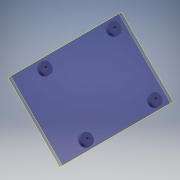
# Autodesk Inventor part: ChassisPrototypeA5
Saved by Autodesk Inventor 2017 (Build 210142000, 142)
## iProperties
Created: 2018-04-24
Part Number: ChassisPrototypeA5
Material: Generic
Document SubType Name: Modeling
Designer: MtgSaber
Mass: 8.35184 g
Surface Area: 62.5115 cm^2
Volume: 8.35184 cm^3
Density: 1 g/cm^3
Appearance: Default
Author: MtgSaber
Autodesk Inventor part; units mm, degrees
ref_plane "YZ Plane" through (0, 0, 0) normal (1, 0, 0) x (0, 1, 0)
ref_plane "Work Plane1" through (108.406, 19.8015, 0) normal (-0.7071068, -0.7071068, 0) x (0, 0, -1)
ref_plane "Work Plane2" through (106.1609, 17.5564, 0) normal (-0.7071068, -0.7071068, 0) x (0, 0, -1)
sketch "Sketch2" plane through (106.1609, 17.5564, 0) normal (-0.7071068, -0.7071068, 0) x (0, 0, -1)
  circle A0 centre (38.989, 24.4983) radius 1.3716 construction
  arc A1 (42.4942, 25.0063) -> (39.497, 28.0035) centre (39.497, 25.0063) ccw construction
  circle A2 centre (38.989, -24.4983) radius 1.3716 construction
  arc A3 (39.497, -28.0035) -> (42.4942, -25.0063) centre (39.497, -25.0063) ccw construction
  circle A4 centre (38.989, 24.4983) radius 1.3716 construction
  circle A5 centre (-18.9992, 24.4983) radius 1.3716 construction
  circle A6 centre (-18.9992, -24.4983) radius 1.3716 construction
  circle A7 centre (38.989, -24.4983) radius 1.3716 construction
  line L0 (-42.4942, 25.0063) -> (-42.4942, -25.0063) construction
  arc A8 (-42.4942, -25.0063) -> (-39.497, -28.0035) centre (-39.497, -25.0063) ccw construction
  line L1 (-39.497, -28.0035) -> (39.497, -28.0035) construction
  arc A9 (39.497, -28.0035) -> (42.4942, -25.0063) centre (39.497, -25.0063) ccw construction
  line L2 (42.4942, -25.0063) -> (42.4942, 25.0063) construction
  arc A10 (42.4942, 25.0063) -> (39.497, 28.0035) centre (39.497, 25.0063) ccw construction
  line L3 (39.497, 28.0035) -> (-39.497, 28.0035) construction
  arc A11 (-39.497, 28.0035) -> (-42.4942, 25.0063) centre (-39.497, 25.0063) ccw construction
  circle A12 centre (38.989, 24.4983) radius 1.3716
  circle A13 centre (38.989, 24.4983) radius 4.5466
  circle A14 centre (38.989, -24.4983) radius 1.3716
  circle A15 centre (38.989, -24.4983) radius 4.5466
  circle A16 centre (-18.9992, -24.4983) radius 1.3716
  circle A17 centre (-18.9992, -24.4983) radius 4.5466
  circle A18 centre (-18.9992, 24.4983) radius 1.3716
  circle A19 centre (-18.9992, 24.4983) radius 4.5466
  point P0 (0, -62.6529)
  dimension "d5" = 3.175
  constraints: 8 centre point, 8 coincident, 7 equal radius
  measures "d5" radial gap between concentric circles of A5 A19
extrude "Extrusion1" add sketch "Sketch2" along normal blind 3.175
ref_plane "Work Plane3" through (127.2196, 3.2509, 0) normal (0, 0, 1) x (-0.7071068, -0.7071068, 0)
sketch "Sketch3" plane through (127.2196, 3.2509, 0) normal (0, 0, 1) x (-0.7071068, -0.7071068, 0)
  line L0 (7.9502, -54.0512) -> (7.9502, -44.958) construction
  line L1 (7.9502, -5.0546) -> (7.9502, 4.0386) construction
  line L2 (7.9502, -54.0512) -> (7.9502, -44.958) construction
  line L3 (7.9502, -54.0512) -> (7.9502, 4.0386) construction
  line L4 (41.241, -25.0063) -> (7.9502, -58.2971) construction
  line L5 (41.241, -25.0063) -> (7.9502, 8.2845) construction
  circle A0 centre (32.2607, -25.0063) radius 2.0574
  arc A1 (36.7508, -29.4964) -> (36.7508, -20.5162) centre (32.2607, -25.0063) ccw
  line L6 (7.9502, -25.0063) -> (55.6437, -25.0063) construction
  circle A2 centre (23.2805, -33.9866) radius 2.0574
  circle A3 centre (23.2805, -33.9866) radius 6.35 construction
  circle A4 centre (14.3002, -7.0458) radius 2.0574
  arc A5 (18.7903, -2.5557) -> (14.3002, -0.6958) centre (14.3002, -7.0458) ccw
  circle A6 centre (23.2805, -16.026) radius 2.0574
  circle A7 centre (23.2805, -16.026) radius 6.35 construction
  circle A8 centre (14.3002, -42.9668) radius 2.0574
  arc A9 (14.3002, -49.3168) -> (18.7903, -47.4569) centre (14.3002, -42.9668) ccw
  circle A10 centre (14.3002, -25.0063) radius 2.0574 construction
  circle A11 centre (14.3002, -25.0063) radius 6.35 construction
  line L7 (7.9502, -42.9668) -> (7.9502, -7.0458)
  line L8 (18.7903, -2.5557) -> (36.7508, -20.5162)
  line L9 (36.7508, -29.4964) -> (18.7903, -47.4569)
  arc A12 (16.3576, -20.8915) -> (12.2428, -20.8915) centre (14.3002, -20.8915) ccw
  line L10 (14.3002, -42.9668) -> (14.3002, -7.0458) construction
  arc A13 (12.2428, -29.1211) -> (16.3576, -29.1211) centre (14.3002, -29.1211) ccw
  arc A14 (18.415, -27.0637) -> (18.415, -22.9489) centre (18.415, -25.0063) ccw
  line L11 (16.3576, -27.0637) -> (18.415, -27.0637)
  line L12 (16.3576, -22.9489) -> (18.415, -22.9489)
  line L13 (16.3576, -27.0637) -> (16.3576, -29.1211)
  line L14 (16.3576, -22.9489) -> (16.3576, -20.8915)
  line L15 (12.2428, -20.8915) -> (12.2428, -29.1211)
  line L16 (14.3002, -49.3168) -> (7.9502, -49.3168)
  line L17 (7.9502, -42.9668) -> (7.9502, -49.3168)
  line L18 (14.3002, -0.6958) -> (7.9502, -0.6958)
  line L19 (7.9502, -0.6958) -> (7.9502, -7.0458)
  point P0 (92.2566, -87.6592)
  dimension "d8" = 45
  dimension "d9" = 4.1148
  dimension "d10" = 12.7
  dimension "d11" = 4.1148
  dimension "d12" = 12.7
  dimension "d13" = 4.1148
  dimension "d14" = 12.7
  dimension "d15" = 4.1148
  dimension "d16" = 12.7
  dimension "d19" = 4.1148
  dimension "d20" = 12.7
  dimension "d21" = 4.1148
  dimension "d22" = 12.7
  dimension "d23" = 4.1148
  dimension "d24" = 4.1148
  dimension "d25" = 4.1148
  constraints: 32 end point, 15 centre point, 13 tangent, 12 point on circle, 10 point on line, 7 equal radius, 6 coincident, 4 parallel, 3 vertical, 2 horizontal, 2 perpendicular, 12 other
  measures "d8" angle to the sketch x axis of L4
  measures "d9" diameter of A0
  measures "d10" diameter of A1
  measures "d11" diameter of A2
  measures "d12" diameter of A3
  measures "d13" diameter of A4
  measures "d14" diameter of A5
  measures "d15" diameter of A6
  measures "d16" diameter of A7
  measures "d19" diameter of A8
  measures "d20" diameter of A9
  measures "d21" diameter of A10
  measures "d22" diameter of A11
  measures "d23" diameter of A12
  measures "d24" diameter of A13
  measures "d25" diameter of A14
extrude "Extrusion2" add sketch "Sketch3" along normal mid plane 4.7625
sketch "Sketch4" plane through (88.838, 34.8793, 18.9992) normal (0.7071068, 0.7071068, 0) x (-0.7071068, 0.7071068, 0)
  line L0 (-48.8088, -16.6179) -> (-0.1878, -16.6179) construction
  line L1 (-0.1878, -21.3804) -> (-48.8088, -21.3804) construction
  circle A0 centre (0, -57.9882) radius 1.3716 construction
  circle A1 centre (0, -57.9882) radius 4.5466 construction
  circle A2 centre (-48.9966, -57.9882) radius 1.3716 construction
  circle A3 centre (-48.9966, -57.9882) radius 4.5466 construction
  circle A4 centre (-48.9966, 0) radius 1.3716 construction
  circle A5 centre (-48.9966, 0) radius 4.5466 construction
  circle A6 centre (0, 0) radius 1.3716 construction
  circle A7 centre (0, 0) radius 4.5466 construction
  line L2 (-48.8088, -18.9992) -> (-0.1878, -18.9992) construction
  line L3 (0, 0) -> (-14.9733, -18.9992) construction
  circle A8 centre (0, -57.9882) radius 1.3716 construction
  line L4 (-14.9733, -18.9992) -> (0, -57.9882) construction
  line L5 (-48.9966, -57.9882) -> (-34.0233, -18.9992) construction
  line L6 (-34.0233, -18.9992) -> (-48.9966, 0) construction
  line L7 (-24.4983, -21.3804) -> (-24.4983, -16.6179) construction
  line L8 (-51.9914, -13.4429) -> (-51.9914, -24.5554)
  line L9 (2.9872, -24.5554) -> (2.9872, -13.4429)
  circle A9 centre (0, 0) radius 4.5466 construction
  line L10 (-4.2676, -1.568) -> (-13.6263, -13.4429)
  line L11 (-0.5271, -4.5159) -> (-7.5625, -13.4429)
  line L12 (0.8344, -53.5188) -> (-10.2887, -24.5554)
  line L13 (-3.6115, -55.2262) -> (-15.3903, -24.5554)
  line L14 (-45.3851, -55.2262) -> (-33.6063, -24.5554)
  line L15 (-49.831, -53.5188) -> (-38.7079, -24.5554)
  circle A10 centre (-48.9966, 0) radius 4.5466 construction
  line L16 (-44.729, -1.568) -> (-35.3703, -13.4429)
  line L17 (-48.4695, -4.5159) -> (-41.4341, -13.4429)
  arc A11 (-4.2676, -1.568) -> (-0.5271, -4.5159) centre (0, 0) ccw
  circle A12 centre (-48.9966, 0) radius 1.3716 construction
  arc A13 (-48.4695, -4.5159) -> (-44.729, -1.568) centre (-48.9966, 0) ccw
  circle A14 centre (-48.9966, -57.9882) radius 1.3716 construction
  arc A15 (-45.3851, -55.2262) -> (-49.831, -53.5188) centre (-48.9966, -57.9882) ccw
  arc A16 (0.8344, -53.5188) -> (-3.6115, -55.2262) centre (0, -57.9882) ccw
  line L18 (2.9872, -13.4429) -> (-7.5625, -13.4429)
  line L19 (-13.6263, -13.4429) -> (-35.3703, -13.4429)
  line L20 (-41.4341, -13.4429) -> (-51.9914, -13.4429)
  line L21 (-51.9914, -24.5554) -> (-38.7079, -24.5554)
  line L22 (-33.6063, -24.5554) -> (-15.3903, -24.5554)
  line L23 (-10.2887, -24.5554) -> (2.9872, -24.5554)
  line L24 (-0.1878, -21.3804) -> (-0.1878, -16.6179) construction
  line L25 (-48.8088, -21.3804) -> (-48.8088, -16.6179) construction
  point P0 (38.1546, -18.9992)
  point P1 (-42.4588, -16.6179)
  point P2 (-6.5378, -16.6179)
  point P3 (-6.5378, -21.3804)
  point P4 (-42.4588, -21.3804)
  dimension "d28" = 19.05
  dimension "d29" = 9.525
  dimension "d34" = 2.3813
  dimension "d35" = 2.3813
  dimension "d36" = 2.3813
  dimension "d37" = 2.3813
  dimension "d38" = 2.3813
  dimension "d39" = 2.3813
  dimension "d40" = 2.3813
  dimension "d41" = 2.3813
  dimension "d42" = 3.175
  dimension "d43" = 3.175
  dimension "d44" = 3.175
  dimension "d45" = 3.1826
  constraints: 44 end point, 21 parallel, 18 point on circle, 4 centre point, 4 coincident, 4 collinear, 4 midpoint, 3 horizontal, 3 perpendicular, 2 point on line, 2 other
  measures "d28" distance of L5.end L3.end
  measures "d29" distance from line of L7 L3.end
  measures "d34" distance between parallel lines of L6 L16
  measures "d35" distance between parallel lines of L14 L5
  measures "d36" distance between parallel lines of L6 L17
  measures "d37" distance between parallel lines of L5 L15
  measures "d38" distance between parallel lines of L4 L13
  measures "d39" distance between parallel lines of L4 L12
  measures "d40" distance between parallel lines of L3 L11
  measures "d41" distance between parallel lines of L3 L10
  measures "d42" distance between parallel lines of L1 L22
  measures "d43" distance between parallel lines of L19 L0
  measures "d44" distance between parallel lines of L24 L9
  measures "d45" distance between parallel lines of L25 L8
extrude "Extrusion3" add sketch "Sketch4" against normal up to surface (3.175 mm away)
fillet "Fillet1" radius 3.175 12 edges at (112.7261, 8.7462, 5.5562) (97.3507, 24.1215, 5.5562) (98.5981, 22.8742, -5.5563) (111.4787, 9.9935, -5.5563) (115.0861, 6.3861, -5.5563) (117.0138, 4.4585, 5.5562) (93.063, 28.4093, 5.5563) (94.9907, 26.4816, -5.5562) (85.6032, 35.8691, 5.5563) (85.6032, 35.8691, -5.5562) (124.479, -3.0067, -5.5563) (124.479, -3.0067, 5.5562)
fillet "Fillet2" radius 3.175 2 edges at (121.106, -1.8788, 0) (86.7257, 32.5015, 0)
body "Solid1"
